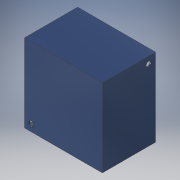
# Autodesk Inventor part: fixaçãoChaveGeral2
Saved by Autodesk Inventor 2019 (Build 230136000, 136)
## iProperties
Created: 2020-05-16
Part Number: fixaçãoChaveGeral2
Material: Genérico
Document SubType Name: Modeling
Designer: eliane
Density: 1 g/cm^3
Appearance: Padrão
Author: eliane
Autodesk Inventor part; units mm, degrees
ref_plane "YZ Plane" through (0, 0, 0) normal (1, 0, 0) x (0, 1, 0)
ref_plane "XZ Plane" through (0, 0, 0) normal (0, 1, 0) x (-1, 0, 0)
ref_plane "XY Plane" through (0, 0, 0) normal (0, 0, 1) x (1, 0, 0)
sketch "Esboço1" plane through (0, 0, 0) normal (1, 0, 0) x (0, 1, 0)
  line L0 (15.0377, 17.4053) -> (-74.9623, 17.4053)
  line L1 (-74.9623, 17.4053) -> (-74.9623, -42.5947)
  line L2 (-74.9623, -42.5947) -> (15.0377, -42.5947)
  line L3 (15.0377, -42.5947) -> (15.0377, 17.4053)
  line L4 (15.0377, -42.5947) -> (15.0377, -34.5947) construction
  line L5 (15.0377, -34.5947) -> (7.0377, -34.5947) construction
  circle A0 centre (7.0377, -34.5947) radius 3 construction
  circle A1 centre (7.0377, -34.5947) radius 3
  point P0 (0, 0)
  dimension "d0" = 90
  dimension "d1" = 60
  dimension "d2" = 8
  dimension "d3" = 8
  dimension "d4" = 6
  constraints: 12 end point, 2 centre point, 2 coincident, 2 parallel, 2 perpendicular, 1 concentric, 1 horizontal, 1 point on line
  measures "d0" distance of L2.end L1.end
  measures "d1" distance of L1.end L0.end
  measures "d2" distance of L2.end L4.end
  measures "d3" distance of L4.end L5.end
  measures "d4" diameter of A0
extrude "Extrusão1" add sketch "Esboço1" along normal blind 1.5
sketch "Esboço2" plane through (0, -74.9623, 17.4053) normal (0, 0, 1) x (1, 0, 0)
  line L0 (1.5, 90) -> (1.5, 0) projected
  line L1 (1.5, 90) -> (-88.5, 90)
  line L2 (-88.5, 90) -> (-88.5, 0)
  line L3 (-88.5, 0) -> (1.5, 0)
  line L4 (1.5, 0) -> (1.5, 90)
  line L5 (-88.5, 0) -> (-80.5, 0) construction
  line L6 (-80.5, 0) -> (-80.5, 8) construction
  line L7 (-80.5, 8) -> (-88.5, 8) construction
  line L8 (-88.5, 8) -> (-88.5, 0) construction
  circle A0 centre (-80.5, 8) radius 3
  point P0 (0, 74.9623)
  dimension "d7" = 90
  dimension "d8" = 8
  dimension "d9" = 8
  dimension "d10" = 6
  constraints: 16 end point, 4 parallel, 2 horizontal, 2 perpendicular, 1 centre point, 1 coincident
  measures "d7" distance of L3.end L2.end
  measures "d8" distance of L7.end L6.end
  measures "d9" distance of L6.end L5.end
  measures "d10" diameter of A0
extrude "Extrusão2" add sketch "Esboço2" along normal blind 1.5
sketch "Esboço3" plane through (-88.5, 15.0377, 17.4053) normal (0, 1, 0) x (1, 0, 0)
  line L0 (88.5, 0) -> (88.5, 60) projected
  line L1 (88.5, 0) -> (0, 0)
  line L2 (0, 0) -> (0, 60)
  line L3 (0, 60) -> (88.5, 60)
  line L4 (88.5, 60) -> (88.5, 0)
  point P0 (88.5, 17.4053)
  dimension "d13" = 88.5
  constraints: 8 end point, 2 parallel, 1 horizontal, 1 perpendicular
  measures "d13" distance of L2.end L3.end
extrude "Extrusão3" add sketch "Esboço3" against normal blind 1.5
sketch "Esboço4" plane through (-88.5, -74.9623, 17.4053) normal (0, -1, 0) x (1, 0, 0)
  line L0 (0, 0) -> (88.5, 0) projected
  line L1 (0, 0) -> (0, -60) projected
  line L2 (88.5, 0) -> (0, 0)
  line L3 (0, 0) -> (0, -60)
  line L4 (0, -60) -> (88.5, -60)
  line L5 (88.5, -60) -> (88.5, 0)
  point P0 (88.5, -17.4053)
  constraints: 8 end point, 2 parallel, 1 horizontal, 1 perpendicular
extrude "Extrusão4" add sketch "Esboço4" against normal blind 1.5
sketch "Esboço5" plane through (-88.5, -74.9623, -42.5947) normal (0, -1, 0) x (1, 0, 0)
  line L0 (0, 61.5) -> (90, 61.5) construction
  line L1 (12.3128, 61.5) -> (6.3128, 61.5) construction
  line L2 (6.3128, 61.5) -> (6.3128, 54.0789) construction
  line L3 (6.3128, 54.0789) -> (12.3128, 54.0789) construction
  line L4 (12.3128, 54.0789) -> (12.3128, 61.5) construction
  point P0 (88.5, 42.5947)
  dimension "d18" = 6
  constraints: 8 end point, 2 parallel, 1 horizontal, 1 perpendicular, 1 point on line
  measures "d18" distance of L3.end L2.end
hole "Furo1" at (-76.1872, -74.9623, 11.4842) at (-82.1872, -74.9623, 11.4842) direction (0, 1, 0) diameter 2.5 depth 1.5 tip angle 118
sketch "Esboço6" plane through (-88.5, -74.9623, -42.5947) normal (0, -1, 0) x (1, 0, 0)
  circle A0 centre (12.3128, 54.0789) radius 1.25 construction
